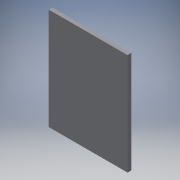
# Autodesk Inventor part: tela
Saved by Autodesk Inventor 2016 (Build 200138000, 138)
## iProperties
Created: 2017-06-05
Part Number: tela
Material: Genérico
Document SubType Name: Modeling
Designer: Fabio
Density: 1 g/cm^3
Appearance: Padrão
Author: Fabio
Autodesk Inventor part; units mm, degrees
ref_plane "YZ Plane" through (0, 0, 0) normal (1, 0, 0) x (0, 1, 0)
ref_plane "XZ Plane" through (0, 0, 0) normal (0, 1, 0) x (-1, 0, 0)
ref_plane "XY Plane" through (0, 0, 0) normal (0, 0, 1) x (1, 0, 0)
sketch "Esboço1" plane through (0, 0, 0) normal (0, 1, 0) x (-1, 0, 0)
  line L0 (127.6443, 137.7783) -> (-125.3557, 137.7783)
  line L1 (-125.3557, 137.7783) -> (-125.3557, -188.2217)
  line L2 (-125.3557, -188.2217) -> (127.6443, -188.2217)
  line L3 (127.6443, -188.2217) -> (127.6443, 137.7783)
  point P0 (0, 0)
  dimension "d0" = 326
  dimension "d1" = 253
  constraints: 8 end point, 2 parallel, 1 horizontal, 1 perpendicular
  measures "d0" distance between parallel lines of L0 L2
  measures "d1" distance between parallel lines of L1 L3
extrude "Extrusão1" add sketch "Esboço1" along normal blind 12
sketch "Esboço2" plane through (0, 12, 0) normal (0, 1, 0) x (1, 0, 0)
  line L0 (-115.6443, -128.7783) -> (113.3557, -128.7783)
  line L1 (113.3557, -128.7783) -> (113.3557, 179.2217)
  line L2 (113.3557, 179.2217) -> (-115.6443, 179.2217)
  line L3 (-115.6443, 179.2217) -> (-115.6443, -128.7783)
  line L4 (-127.6443, -137.7783) -> (125.3557, -137.7783) projected
  line L5 (125.3557, 188.2217) -> (-127.6443, 188.2217) projected
  line L6 (-127.6443, 188.2217) -> (-127.6443, -137.7783) projected
  line L7 (125.3557, -137.7783) -> (125.3557, 188.2217) projected
  point P0 (0, 0)
  dimension "d4" = 9
  dimension "d5" = 9
  dimension "d6" = 12
  dimension "d7" = 12
  constraints: 8 end point, 2 parallel, 1 horizontal, 1 perpendicular
  measures "d4" distance between parallel lines of L0 L4
  measures "d5" distance between parallel lines of L5 L2
  measures "d6" distance between parallel lines of L6 L3
  measures "d7" distance between parallel lines of L1 L7
extrude "Extrusão2" cut sketch "Esboço2" against normal blind 2 contours L3 L2 L1 L0
